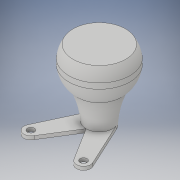
# Autodesk Inventor part: 25 deurknop
Saved by Autodesk Inventor 2019 (Build 230136000, 136)
## iProperties
Created: 2021-04-27
Part Number: 25 deurknop
Material: Generic
Document SubType Name: Modeling
Designer: daanswinters
Density: 1 g/cm^3
Appearance: Default
Author: daanswinters
Autodesk Inventor part; units mm, degrees
ref_plane "YZ Plane" through (0, 0, 0) normal (1, 0, 0) x (0, 1, 0)
ref_plane "XZ Plane" through (0, 0, 0) normal (0, 1, 0) x (-1, 0, 0)
ref_plane "XY Plane" through (0, 0, 0) normal (0, 0, 1) x (1, 0, 0)
sketch "Sketch1" plane through (0, 0, 0) normal (0, 0, 1) x (1, 0, 0)
  line L0 (0, 0) -> (0, 40)
  line L1 (0, 40) -> (15, 40)
  line L2 (0, 40) -> (15, 40) construction
  line L3 (17.3638, 33.076) -> (17.3638, 29.9583)
  arc A0 (11.9847, 19.4992) -> (7.5, 0) centre (59.0045, -1.5803) ccw
  arc A1 (11.9847, 19.4992) -> (15, 40) centre (1.4748, 31.5172) ccw
  line L4 (7.5, 0) -> (0, 0)
  dimension "d0" = 40
  dimension "d2" = 15
  dimension "d3" = 0
  dimension "d5" = 90
  dimension "d6" = 7.5
  dimension "d8" = 15.9652
  dimension "d10" = 17.3638
  dimension "d11" = 6.924
  dimension "d12" = 2.3638
  dimension "d13" = 5.3791
  dimension "d14" = 51.5287
  constraints: 10 end point, 6 point on circle, 2 centre point, 2 horizontal, 2 perpendicular, 1 vertical
  measures "d0" distance of L0.start L0.end
  measures "d2" distance of L0.end L1.end
  measures "d3" distance between parallel lines of L1 L2
  measures "d5" angle of L1 L3
  measures "d6" distance of L0.start L4.start
  measures "d8" radius of A1
  measures "d10" distance between parallel lines of L0 L3
  measures "d11" distance from line of L3.start L2
  measures "d12" distance from line of L2.end L3
  measures "d13" distance from line of A0.start L3
  measures "d14" radius of A0
revolve "Revolution1" add sketch "Sketch1" angle 360 about axis through (0, 0, 0) along (0, 1, 0) contours L0 L1 A1 L3 A0 L4
sketch "Sketch2" plane through (0, 0, 0) normal (0, -1, 0) x (1, 0, 0)
  point P0 (0, 0)
sketch "Sketch3" plane through (0, 0, 0) normal (0, -1, 0) x (1, 0, 0)
  line L0 (0, 0) -> (-15, 0) construction
  line L1 (-15, 0) -> (-15, 24) construction
  circle A0 centre (-15, 24) radius 2
  circle A1 centre (15, 24) radius 2
  circle A2 centre (15, 24) radius 4
  circle A3 centre (-15, 24) radius 4
  arc A4 (-7.5, 0) -> (6.8027, -3.158) centre (0, 0) ccw
  circle A5 centre (0, 0) radius 7.5 projected
  line L2 (18.6281, 22.3158) -> (6.8027, -3.158)
  line L3 (-18.6281, 22.3158) -> (-6.8027, -3.158)
  line L4 (11.3719, 25.6842) -> (0, 7.5)
  line L5 (-11.3719, 25.6842) -> (0, 7.5)
  dimension "d15" = 15
  dimension "d16" = 24
  dimension "d17" = 4
  dimension "d18" = 4
  dimension "d19" = 30
  dimension "d20" = 24
  dimension "d21" = 2
  dimension "d22" = 2
  dimension "d23" = 7.119
  dimension "d24" = 56.922
  dimension "d25" = 3.9767
  constraints: 12 end point, 9 point on circle, 5 centre point, 4 tangent, 2 coincident, 1 horizontal, 1 midpoint, 1 perpendicular
  measures "d15" distance of L0.start L0.end
  measures "d16" distance of L0.end L1.end
  measures "d17" diameter of A0
  measures "d18" diameter of A1
  measures "d19" distance of A0.centre A1.centre
  measures "d20" vertical distance of L0.start A1.centre
  measures "d21" radial gap between concentric circles of A1 A2
  measures "d22" radial gap between concentric circles of A0 A3
  measures "d23" angle of L4 L2
  measures "d24" angle of L5 L2
  measures "d25" distance from line of L0.start L4
extrude "Extrusion1" add sketch "Sketch3" against normal blind 2 contours A2 | A2 L2 A5 L4 | A5 A4 L3 A3 L5 | A3
body "Solid1"
